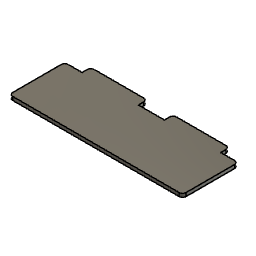
VFD_NTP_CLOCK_PLATE_F_V1.0 v3 (Autodesk Fusion 360 design; units mm, degrees)
Autodesk Fusion 360 part; units mm, degrees
sketch "スケッチ1" plane through (0, 0, 0) normal (0, 1, 0) x (1, 0, 0)
  line L0 (-48, 0) -> (48, 0)
  line L1 (-50.0166, 2) -> (-50.0166, 30)
  line L2 (-48, 32) -> (-40, 32)
  line L3 (-40, 32) -> (-40, 35)
  line L4 (-38, 37) -> (-9.5, 37)
  line L5 (50, 2) -> (50, 30)
  line L6 (48, 32) -> (40, 32)
  line L7 (40, 32) -> (40, 35)
  line L8 (38, 37) -> (9.5, 37)
  line L9 (-7.5, 32) -> (7.5, 32)
  arc A0 (-38, 37) -> (-40, 35) centre (-38, 35) ccw
  line L10 (-7.5, 35.0262) -> (-7.5, 32)
  line L11 (7.4996, 35.0262) -> (7.5, 32)
  arc A1 (-48, 32) -> (-50.0166, 30) centre (-48, 29.9833) ccw
  arc A2 (-7.5, 35.0262) -> (-9.5, 37) centre (-9.5, 34.9998) ccw
  arc A3 (9.5, 37) -> (7.4996, 35.0262) centre (9.5, 34.9994) ccw
  arc A4 (40, 35) -> (38, 37) centre (38, 35) ccw
  arc A5 (50, 30) -> (48, 32) centre (48, 30) ccw
  arc A6 (48, 0) -> (50, 2) centre (48, 2) ccw
  arc A7 (-50.0166, 2) -> (-48, 0) centre (-48.0165, 2) ccw
  dimension "d1" = 96
  dimension "d2" = 28
  dimension "d3" = 8
  dimension "d4" = 28.5
  dimension "d5" = 28
  dimension "d6" = 8
  dimension "d7" = 28.5
  constraint horizontal L0
  constraint perpendicular L0 L1
  constraint horizontal L2
  constraint perpendicular L2 L3
  constraint perpendicular L3 L4
  constraint perpendicular L0 L5
  constraint horizontal L6
  constraint perpendicular L6 L7
  constraint horizontal L8
  constraint horizontal L9
  constraint tangent L4 A0
  constraint perpendicular L9 L10
  constraint tangent L2 A1
  constraint tangent L4 A2
  constraint tangent L8 A3
  constraint tangent L8 A4
  constraint tangent L6 A5
  constraint tangent L5 A6
  constraint tangent L1 A7
  measures "d1" distance of L0.start L0.end
  measures "d2" distance of L1.start L1.end
  measures "d3" distance of L2.start L2.end
  measures "d4" distance of L4.start L4.end
  measures "d5" distance of L5.start L5.end
  measures "d6" distance of L6.start L6.end
  measures "d7" distance of L8.start L8.end
extrude "押し出し1" add sketch "スケッチ1" along normal blind 2
